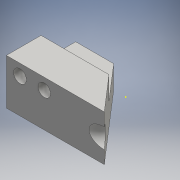
# Autodesk Inventor part: 240510_3Dsketch01
Saved by Autodesk Inventor 2016 (Build 200138000, 138)
## iProperties
Created: 2024-05-10
Part Number: 240510_3Dsketch01
Material: 일반
Document SubType Name: Modeling
Designer: pc
Density: 1 g/cm^3
Appearance: 기본값
Author: pc
Autodesk Inventor part; units mm, degrees
ref_plane "YZ Plane" through (0, 0, 0) normal (1, 0, 0) x (0, 1, 0)
ref_plane "XZ Plane" through (0, 0, 0) normal (0, 1, 0) x (-1, 0, 0)
ref_plane "XY Plane" through (0, 0, 0) normal (0, 0, 1) x (1, 0, 0)
sketch "스케치1" plane through (0, 0, 0) normal (0, 0, 1) x (1, 0, 0)
  line L0 (-109.2986, 75.8401) -> (105.1639, 75.8401)
  line L1 (105.1639, 75.8401) -> (105.1639, -75.9568)
  line L2 (105.1639, -75.9568) -> (-109.2986, -75.9568)
  line L3 (-109.2986, -75.9568) -> (-109.2986, 75.8401)
  point P0 (0, 0)
  constraints: 8 end point, 2 parallel, 1 horizontal, 1 perpendicular
extrude "돌출1" add sketch "스케치1" along normal blind 100
sketch "스케치2" plane through (0, 0, 100) normal (0, 0, 1) x (1, 0, 0)
  line L0 (-109.2986, -75.9568) -> (105.1639, -75.9568) projected
  line L1 (-26.2714, 75.9875) -> (105.1639, -75.9568)
  line L2 (105.1639, -75.9568) -> (105.1639, 75.9875)
  line L3 (105.1639, 75.9875) -> (-26.2714, 75.9875)
  point P0 (0, 0)
  constraints: 6 end point, 2 perpendicular
extrude "돌출2" cut sketch "스케치2" against normal blind 100
sketch "스케치3" plane through (-109.2986, 75.8401, 100) normal (0, 1, 0) x (1, 0, 0)
  point P0 (109.2986, 100)
sketch "스케치4" plane through (0, 0, 100) normal (0, 0, 1) x (1, 0, 0)
  line L0 (-109.2986, -75.9568) -> (-109.2986, 75.8401) projected
  line L1 (-109.2986, 75.8401) -> (-109.2986, -0.0583)
  line L2 (-26.1439, 75.8401) -> (105.1639, -75.9568) projected
  line L3 (39.51, -0.0583) -> (-26.1439, 75.8401)
  line L4 (-26.1439, 75.8401) -> (-109.2986, 75.8401)
  line L5 (-109.2986, -0.0583) -> (39.51, -0.0583)
  point P0 (0, 0)
  constraints: 8 end point, 2 midpoint, 1 collinear, 1 horizontal, 1 perpendicular
extrude "돌출3" cut sketch "스케치4" against normal blind 50
sketch "스케치5" plane through (-109.2986, -0.0583, 100) normal (0, 1, 0) x (1, 0, 0)
  circle A0 centre (83.0272, 24.3451) radius 13.7114
  circle A1 centre (29.8194, 24.3451) radius 14.1089
  point P0 (109.2986, 100)
  constraints: 2 centre point
extrude "돌출4" cut sketch "스케치5" against normal blind 80
sketch "스케치6" plane through (105.1639, -75.9568, 100) normal (0.7563, 0.6542, 0) x (0, 0, -1)
  circle A0 centre (50, 0.3021) radius 21.6251
  point P0 (100, 126.2468)
  constraints: 1 centre point
extrude "돌출5" cut sketch "스케치6" against normal blind 80
